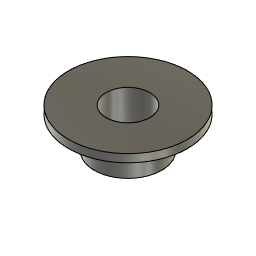
Quark MFR Washer (Autodesk Fusion 360 design; units mm, degrees)
Autodesk Fusion 360 part; units mm, degrees
sketch "Sketch1" plane through (0, 0, 0) normal (0, 0, 1) x (1, 0, 0)
  circle A0 centre (0, 0) radius 1.7
  circle A1 centre (0, 0) radius 1.1
  dimension "d1" = 2.2
  dimension "d2" = 3.4
  constraint coincident A0.centre A1.centre
  constraint concentric A0 A1
  measures "d1" diameter of A1
  measures "d2" diameter of A0
extrude "Extrude1" add sketch "Sketch1" against normal blind 1.6
sketch "Sketch2" plane through (0, 0, 0) normal (0, 0, 1) x (-1, 0, 0)
  circle A0 centre (0, 0) radius 1.1
  circle A1 centre (0, 0) radius 1.7
  circle A2 centre (0, 0) radius 3
  dimension "d5" = 6
  measures "d5" diameter of A2
extrude "Extrude2" add sketch "Sketch2" along normal blind 0.4 contours A1 | A2
